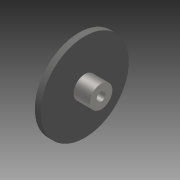
# Autodesk Inventor part: Hitec HS-225MG gear 2
Saved by Autodesk Inventor 2017 SP1 (Build 210196100, 196)
## iProperties
Created: 2018-01-04
Part Number: Hitec HS-225MG gear 2
Material: Generic
Document SubType Name: Modeling
Designer: JT
Density: 1 g/cm^3
Appearance: Default
Author: JT
Autodesk Inventor part; units mm, degrees
ref_plane "YZ Plane" through (0, 0, 0) normal (1, 0, 0) x (0, 1, 0)
ref_plane "XZ Plane" through (0, 0, 0) normal (0, 1, 0) x (-1, 0, 0)
ref_plane "XY Plane" through (0, 0, 0) normal (0, 0, 1) x (1, 0, 0)
sketch "Sketch1" plane through (0, 0, 0) normal (0, 0, 1) x (1, 0, 0)
  line L0 (0, 0) -> (0, 5.9)
  line L1 (0, 5.9) -> (0.8, 5.9)
  line L2 (0.8, 5.9) -> (0.8, 1.5)
  line L3 (0.8, 1.5) -> (3, 1.5)
  line L4 (3, 1.5) -> (3, 0)
  line L5 (3, 0) -> (0, 0)
  dimension "d0" = 0.8
  dimension "d1" = 3
  dimension "d2" = 11.8
  dimension "d3" = 3
  constraints: 12 end point, 5 perpendicular, 1 vertical
  measures "d0" distance between parallel lines of L2 L0
  measures "d1" distance between parallel lines of L4 L0
  measures "d2" diameter of L1 L5
  measures "d3" diameter of L3 L5
revolve "Revolution1" add sketch "Sketch1" angle 360 about axis through (3, 0, 0) along (-1, 0, 0)
hole "Hole1" at (3, 0, 0) direction (-1, 0, 0) diameter 1.2 end through all
body "Solid1"
